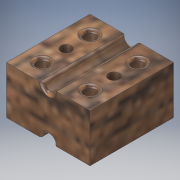
# Autodesk Inventor part: MiddleOfSquareSupport
Saved by Autodesk Inventor 2017 SP1 (Build 210196100, 196)
## iProperties
Created: 2015-12-08
Part Number: MiddleOfSquareSupport
Material: PC/ABS Plastic
Document SubType Name: Modeling
Designer: steele
Density: 0.357273 g/cm^3
Appearance: White Ash - Java
Author: steele
Autodesk Inventor part; units mm, degrees
ref_plane "YZ Plane" through (0, 0, 0) normal (1, 0, 0) x (0, 1, 0)
ref_plane "XZ Plane" through (0, 0, 0) normal (0, 1, 0) x (-1, 0, 0)
ref_plane "XY Plane" through (0, 0, 0) normal (0, 0, 1) x (1, 0, 0)
sketch "Sketch1" plane through (0, 0, 0) normal (0, 1, 0) x (-1, 0, 0)
  line L0 (-22.225, 22.225) -> (-22.225, -22.225)
  line L1 (-22.225, -22.225) -> (22.225, -22.225)
  line L2 (22.225, -22.225) -> (22.225, 22.225)
  line L3 (22.225, 22.225) -> (-22.225, 22.225)
  line L4 (-22.225, 22.225) -> (22.225, -22.225) construction
  line L5 (-22.225, -22.225) -> (22.225, 22.225) construction
  point P0 (0, 0)
  dimension "d4" = 44.45
  constraints: 12 end point, 2 midpoint, 2 parallel, 2 perpendicular, 1 vertical
  measures "d4" distance of L0.start L0.end
extrude "Extrusion1" add sketch "Sketch1" along normal blind 25.4
sketch "Sketch3" plane through (-22.225, 0, 22.225) normal (0, 0, 1) x (1, 0, 0)
  line L0 (44.45, 25.4) -> (0, 25.4) construction
  point P0 (22.225, 0)
  point P1 (22.225, 25.4)
  point P2 (22.225, 0)
  constraints: 1 coincident, 1 midpoint
hole "Hole1" at (0, 25.4, 22.225) at (0, 0, 22.225) direction (0, 0, -1) diameter 6.35 end through all
sketch "Sketch4" plane through (0, 25.4, 0) normal (0, 1, 0) x (1, 0, 0)
  line L0 (-22.225, 22.225) -> (-22.225, -22.225) projected
  line L1 (22.225, -22.225) -> (22.225, 22.225) projected
  line L2 (-22.225, -22.225) -> (-3.175, -22.225) projected
  line L3 (3.175, -22.225) -> (22.225, -22.225) projected
  point P0 (0, 0)
  point P1 (-12.7, 0)
  point P2 (12.7, 0)
  dimension "d16" = 9.525
  dimension "d17" = 9.525
  dimension "d25" = 22.225
  dimension "d26" = 22.225
  measures "d16" distance from line of point (-12.7, 0) L0
  measures "d17" distance from line of point (12.7, 0) L1
  measures "d25" distance from line of point (-12.7, 0) L2
  measures "d26" distance from line of L3 point (12.7, 0)
hole "Hole2" at (-12.7, 25.4, 0) at (12.7, 25.4, 0) direction (0, -1, 0) diameter 5.6134 end through all clearance for "Flat Head Machine Screw (82)" size "#10" standard "Ansi Unified Screw Threads"
sketch "Sketch5" plane through (0, 25.4, 0) normal (0, 1, 0) x (1, 0, 0)
  line L0 (-12.7, -12.7) -> (12.7, -12.7) construction
  line L1 (12.7, -12.7) -> (12.7, 12.7) construction
  line L2 (12.7, 12.7) -> (-12.7, 12.7) construction
  line L3 (-12.7, 12.7) -> (-12.7, -12.7) construction
  line L4 (-12.7, -12.7) -> (12.7, 12.7) construction
  line L5 (12.7, -12.7) -> (-12.7, 12.7) construction
  line L6 (-22.225, -22.225) -> (-3.175, -22.225) projected
  line L7 (-22.225, 22.225) -> (-22.225, -22.225) projected
  circle A0 centre (-12.7, -12.7) radius 3.048
  circle A1 centre (12.7, -12.7) radius 3.048
  circle A2 centre (12.7, 12.7) radius 3.048
  circle A3 centre (-12.7, 12.7) radius 3.048
  point P0 (0, 0)
  dimension "d27" = 9.525
  dimension "d28" = 9.525
  dimension "d29" = 6.096
  constraints: 12 end point, 4 centre point, 4 coincident, 3 equal radius, 2 midpoint, 2 parallel, 1 horizontal, 1 perpendicular
  measures "d27" distance between parallel lines of L6 L0
  measures "d28" distance between parallel lines of L7 L3
  measures "d29" diameter of A0
extrude "Extrusion2" cut sketch "Sketch5" against normal through all
fillet "Fillet1" radius 1.5875 4 edges at (-3.175, 25.4, 0) (3.175, 25.4, 0) (0, 22.225, 22.225) (0, 22.225, -22.225)
fillet "Fillet2" radius 1.5875 4 edges at (3.175, 0, 0) (-3.175, 0, 0) (0, 3.175, 22.225) (0, 3.175, -22.225)
fillet "Fillet3" radius 1.5875 4 edges at (9.652, 0, 12.7) (9.652, 0, -12.7) (-15.748, 0, -12.7) (-15.748, 0, 12.7)
fillet "Fillet4" radius 1.5875 4 edges at (-15.748, 25.4, -12.7) (-15.748, 25.4, 12.7) (9.652, 25.4, 12.7) (9.652, 25.4, -12.7)
equation "\"d4\" = baseWidth"
equation "\"d6\" = heightOfMiddleSection"
equation "\"d9\" = bottomHoleDiam"
equation "\"d16\" = edgeToBoltHole"
equation "\"d17\" = edgeToBoltHole"
equation "\"d25\" = 0.5 * baseWidth"
equation "\"d26\" = 0.5 * baseWidth"
equation "\"d27\" = edgeToBoltHole"
equation "\"d28\" = edgeToBoltHole"
equation "\"d29\" = supportHoleDiam"
equation "\"bottomHoleDiam\" = 6.35"
equation "\"baseWidth\" = 44.45"
equation "\"deltaBottomToTop\" = 27.94"
equation "\"d0\" = baseWidth"
equation "\"d1\" = heightOfBottomHole"
equation "\"d2\" = 0"
equation "\"d3\" = bottomHoleDiam"
equation "\"d5\" = 0"
equation "\"height\" = deltaBottomToTop + heightOfBottomHole + heightOfTopHole"
equation "\"topHoleDiam\" = 9.525"
equation "\"edgeToBoltHole\" = -0.25 * bottomHoleDiam + 0.25 * baseWidth"
equation "\"heightOfMiddleSection\" = 25.4"
equation "\"baseLength\" = 44.45"
equation "\"supportHoleDiam\" = 6.096"
equation "\"heightOfBottomHole\" = 9.525"
equation "\"heightOfTopHole\" = 9.525"
body "Solid1"
